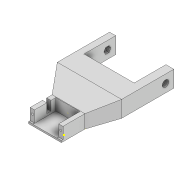
# Autodesk Inventor part: Part5
Saved by Autodesk Inventor 2022 (Build 260153000, 153)
## iProperties
Created: 2021-06-22
Part Number: Part5
Material: Generic
Document SubType Name: Modeling
Designer: Prajwal Patil
Density: 1 g/cm^3
Appearance: Default
Author: Prajwal Patil
Autodesk Inventor part; units mm, degrees
ref_plane "YZ Plane" through (0, 0, 0) normal (1, 0, 0) x (0, 1, 0)
sketch "Sketch1" plane through (0, 0, 0) normal (0, 0, 1) x (1, 0, 0)
  line L0 (-20.399473, 8.732571) -> (20.240527, 8.732571)
  line L1 (20.240527, 8.732571) -> (20.240527, -7.777429)
  line L2 (20.240527, -7.777429) -> (-20.399473, -7.777429)
  line L3 (-20.399473, -7.777429) -> (-20.399473, 8.732571)
  point P0 (0, 0)
  dimension "d0" = 40.64
  dimension "d1" = 16.51
  constraints: 8 end point, 2 parallel, 1 horizontal, 1 perpendicular
  measures "d0" distance of L1.end L2.end
  measures "d1" distance of L0.end L1.end
extrude "Extrusion1" add sketch "Sketch1" against normal blind 27.178
sketch "Sketch2" plane through (0, 0, 0) normal (0, 0, 1) x (1, 0, 0)
  line L0 (20.240527, -7.777429) -> (-20.399473, -7.777429)
  line L1 (-20.399473, -7.777429) -> (-20.399473, -5.491429)
  line L2 (-20.399473, -7.777429) -> (-20.399473, 8.732571)
  line L3 (-20.399473, -5.491429) -> (-15.065473, -5.491429)
  line L4 (-15.065473, -5.491429) -> (-15.065473, -5.745429)
  line L5 (20.240527, -7.777429) -> (20.240527, -5.491429)
  line L6 (20.240527, 8.732571) -> (20.240527, -7.777429)
  line L7 (20.240527, -5.491429) -> (14.906527, -5.491429)
  line L8 (14.906527, -5.491429) -> (14.906527, -5.745429)
  line L9 (-15.065473, -5.745429) -> (14.906527, -5.745429)
  point P0 (0, 0)
  dimension "d4" = 2.286
  dimension "d5" = 5.334
  dimension "d6" = 0.254
  dimension "d7" = 2.286
  dimension "d8" = 5.334
  dimension "d9" = 0.254
  constraints: 14 end point, 2 horizontal, 2 perpendicular, 2 point on line
  measures "d4" distance of L0.end L1.end
  measures "d5" distance of L1.end L3.end
  measures "d6" distance of L3.end L4.end
  measures "d7" distance of L0.start L5.end
  measures "d8" distance of L5.end L7.end
  measures "d9" distance of L7.end L8.end
extrude "Extrusion2" add sketch "Sketch2" along normal blind 2.032
sketch "Sketch3" plane through (0, 0, 0) normal (0, 0, 1) x (1, 0, 0)
  line L0 (-20.399473, 8.732571) -> (-20.399473, -5.491429)
  line L1 (20.240527, 8.732571) -> (-20.399473, 8.732571)
  line L2 (14.906527, -5.745429) -> (-15.065473, -5.745429)
  line L3 (-15.065473, 8.732571) -> (-15.065473, -5.745429)
  line L4 (-15.065473, -5.745429) -> (14.906527, -5.745429)
  line L5 (14.906527, -5.745429) -> (14.906527, 8.732571)
  line L6 (-15.065473, 8.732571) -> (14.906527, 8.732571)
  point P0 (0, 0)
  dimension "d12" = 5.334
  constraints: 8 end point, 2 point on line, 1 collinear, 1 perpendicular
  measures "d12" distance of L0.start L3.start
extrude "Extrusion3" cut sketch "Sketch3" against normal blind 26.416
ref_plane "Work Plane1" through (0, 0, -61.468) normal (0, 0, -1) x (-1, 0, 0)
sketch "Sketch6" plane through (0, 0, -27.178) normal (0, 0, -1) x (-1, 0, 0)
  line L0 (20.399473, -7.777429) -> (-20.240527, -7.777429)
  point P0 (0, 0)
sketch "Sketch8" plane through (0, 0, -61.468) normal (0, 0, -1) x (-1, 0, 0)
  line L0 (0, 12.542354) -> (44.128566, 12.542354)
  line L1 (-20.240527, -7.777429) -> (20.399473, -7.777429)
  line L2 (0.079473, -7.777429) -> (44.128566, -7.777429)
  line L3 (-31.467332, 12.542354) -> (48.234468, 12.542354)
  line L4 (48.234468, 12.542354) -> (48.234468, -7.777429)
  line L5 (48.234468, -7.777429) -> (-31.467332, -7.777429)
  line L6 (-31.467332, -7.777429) -> (-31.467332, 12.542354)
  line L7 (-31.467332, 12.542354) -> (48.234468, 12.542354)
  line L8 (48.234468, 12.542354) -> (48.234468, -7.777429)
  line L9 (48.234468, -7.777429) -> (-31.467332, -7.777429)
  line L10 (-31.467332, -7.777429) -> (-31.467332, 12.542354)
  point P0 (0, 0)
  constraints: 20 end point, 4 parallel, 3 horizontal, 2 perpendicular, 1 midpoint
sketch "Sketch8 outline for Loft1" plane through (0, 0, -61.468) normal (0, 0, -1) x (-1, 0, 0)
  line L0 (48.234468, 12.542354) -> (-31.467332, 12.542354)
  line L1 (48.234468, -7.777429) -> (48.234468, 12.542354)
  line L2 (-31.467332, -7.777429) -> (48.234468, -7.777429)
  line L3 (-31.467332, 12.542354) -> (-31.467332, -7.777429)
loft "Loft1" add profiles "Sketch8 outline for Loft1" section 1 edges at (-0.079473, -7.777429, -27.178) (-20.399473, 0.477571, -27.178) (-0.079473, 8.732571, -27.178) (20.240527, 0.477571, -27.178)
ref_plane "Work Plane2" through (31.467332, -7.777429, -126.238) normal (0, 0, -1) x (-1, 0, 0)
extrude "Extrusion4" add sketch "Sketch8" along normal blind 64.77
sketch "Sketch9" plane through (0, 0, -126.238) normal (0, 0, -1) x (-1, 0, 0)
  line L0 (40.614468, -7.777429) -> (40.614468, 12.542354)
  line L1 (-31.467332, 12.542354) -> (48.234468, 12.542354)
  line L2 (40.614468, 12.542354) -> (-21.615532, 12.542354)
  line L3 (-21.615532, 12.542354) -> (-21.615532, -7.777429)
  line L4 (-20.240527, -7.777429) -> (-31.467332, -7.777429)
  line L5 (-21.615532, -7.777429) -> (40.614468, -7.777429)
  point P0 (0, 0)
  point P1 (48.234468, -7.777429)
  dimension "d27" = 7.62
  dimension "d28" = 62.23
  constraints: 8 end point, 2 perpendicular, 2 point on line
  measures "d27" distance of point (48.234, -7.777) L0.start
  measures "d28" distance of L0.end L2.end
extrude "Extrusion5" cut sketch "Sketch9" against normal blind 39.37
sketch "Sketch10" plane through (21.615532, -7.777429, -126.238) normal (-1, 0, 0) x (0, 0, 1)
  point P0 (126.238, 7.777429)
sketch "Sketch11" plane through (31.467332, -7.777429, -61.468) normal (1, 0, 0) x (0, 0, -1)
  line L0 (64.77, 0) -> (64.77, 20.319783)
  line L1 (64.77, 10.159891) -> (54.356, 10.159891)
  circle A0 centre (54.356, 10.159891) radius 2.54
  circle A1 centre (54.356, 10.159891) radius 4.064
  point P0 (-61.468, 7.777429)
  dimension "d31" = 10.414
  dimension "d32" = 5.08
  dimension "d33" = 8.128
  constraints: 2 centre point, 2 coincident, 2 end point, 1 horizontal, 1 midpoint
  measures "d31" distance of L1.start L1.end
  measures "d32" diameter of A0
  measures "d33" diameter of A1
extrude "Extrusion6" cut sketch "Sketch11" against normal through all contours A0
sketch "Sketch12" plane through (-20.399473, -5.491429, 0) normal (-1, 0, 0) x (0, 0, 1)
  line L0 (-27.178, -2.286) -> (2.032, -2.286) projected
  line L1 (-20.32, -2.286) -> (-15.24, -2.286) construction
  line L2 (-20.32, 2.794) -> (-15.24, 2.794)
  line L3 (-15.24, 2.794) -> (-15.24, 14.224)
  line L4 (-20.32, 2.794) -> (-20.32, 14.224)
  line L5 (-20.32, 14.224) -> (-15.24, 14.224)
  point P0 (0, 5.491429)
  point P1 (-27.178, 14.224)
  dimension "d36" = 6.858
  dimension "d37" = 5.08
  dimension "d39" = 5.08
  constraints: 10 end point, 1 horizontal, 1 point on line
  measures "d36" distance of point (-27.178, 14.224) L4.end
  measures "d37" distance of L1.start L2.start
  measures "d39" distance of L2.start L2.end
extrude "Extrusion7" cut sketch "Sketch12" against normal blind 25.4
sketch "Sketch13" plane through (0, 0, 0) normal (0, 0, 1) x (1, 0, 0)
  line L0 (-15.065473, -5.491429) -> (-20.399473, -5.491429)
  line L1 (-20.399473, -5.491429) -> (-17.605473, -5.491429)
  circle A0 centre (-17.605473, 2.890571) radius 1.27
  line L2 (20.240527, -5.491429) -> (14.906527, -5.491429)
  line L3 (20.240527, -5.491429) -> (17.446527, -5.491429)
  circle A1 centre (17.446527, 2.890571) radius 1.27
  point P0 (0, 0)
  dimension "d42" = 2.794
  dimension "d44" = 2.54
  dimension "d45" = 2.794
  dimension "d47" = 2.54
  constraints: 4 end point, 2 centre point, 2 point on line
  measures "d42" distance of L0.end L1.end
  measures "d44" diameter of A0
  measures "d45" distance of L2.start L3.end
  measures "d47" diameter of A1
extrude "Extrusion8" cut sketch "Sketch13" against normal blind 2.54
sketch "Sketch15" plane through (31.467332, -7.777429, -61.468) normal (1, 0, 0) x (0, 0, -1)
  circle A0 centre (54.356, 10.159891) radius 2.54
  circle A1 centre (54.356, 10.159891) radius 4.064
  point P0 (-61.468, 7.777429)
  dimension "d51" = 8.128
  constraints: 1 centre point, 1 coincident
  measures "d51" diameter of A1
extrude "Extrusion9" cut sketch "Sketch15" against normal blind 3.81 contours A0 | A1
sketch "Sketch16" plane through (21.615532, -7.777429, -126.238) normal (-1, 0, 0) x (0, 0, 1)
  point P0 (126.238, 7.777429)
sketch "Sketch17" plane through (21.615532, -7.777429, -126.238) normal (-1, 0, 0) x (0, 0, 1)
  circle A0 centre (10.414, 10.159891) radius 2.54
  circle A1 centre (10.414, 10.159891) radius 4.064
  point P0 (126.238, 7.777429)
  dimension "d54" = 8.128
  constraints: 1 centre point, 1 coincident
  measures "d54" diameter of A1
extrude "Extrusion10" cut sketch "Sketch17" against normal blind 3.81 contours A0 | A1
sketch "Sketch18" plane through (-40.614468, -7.777429, -126.238) normal (1, 0, 0) x (0, 0, -1)
  circle A0 centre (-10.414, 10.159891) radius 2.54
  line L0 (-8.246516, 6.425305) -> (-12.564505, 6.415502)
  line L1 (-12.564505, 6.415502) -> (-14.731989, 10.150089)
  line L2 (-14.731989, 10.150089) -> (-12.581484, 13.894478)
  line L3 (-12.581484, 13.894478) -> (-8.263495, 13.904281)
  line L4 (-8.263495, 13.904281) -> (-6.096011, 10.169694)
  line L5 (-6.096011, 10.169694) -> (-8.246516, 6.425305)
  point P0 (-126.238, 7.777429)
  constraints: 12 end point, 2 coincident, 13 other
extrude "Extrusion12" cut sketch "Sketch18" against normal blind 3.81
equation "\"d48\" = d47"
body "Solid1"
